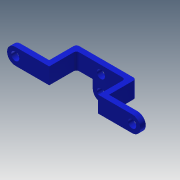
# Autodesk Inventor part: tahlo6
Saved by Autodesk Inventor 2015 (Build 190159000, 159)
## iProperties
Created: 2013-03-23
Part Number: tahlo6
Material: Generic
Document SubType Name: Modeling
Designer: idle-rug
Density: 1 g/cm^3
Appearance: Default
Author: idle-rug
Autodesk Inventor part; units mm, degrees
ref_plane "YZ Plane" through (0, 0, 0) normal (1, 0, 0) x (0, 1, 0)
ref_plane "XZ Plane" through (0, 0, 0) normal (0, 1, 0) x (-1, 0, 0)
ref_plane "XY Plane" through (0, 0, 0) normal (0, 0, 1) x (1, 0, 0)
sketch "Sketch1" plane through (0, 0, 0) normal (0, 1, 0) x (-1, 0, 0)
  line L0 (11, 3) -> (-11, 3)
  line L1 (-11, 3) -> (-11, -3)
  line L2 (-11, -3) -> (11, -3)
  line L3 (11, -3) -> (11, 3)
  line L4 (11, 3) -> (-11, -3) construction
  line L5 (-11, 3) -> (11, -3) construction
  point P0 (0, 0)
  dimension "d0" = 22
  dimension "d1" = 6
  constraints: 12 end point, 2 midpoint, 2 parallel, 1 horizontal, 1 perpendicular
  measures "d0" distance of L2.end L1.end
  measures "d1" distance of L1.end L0.end
extrude "Extrusion1" add sketch "Sketch1" along normal blind 2
sketch "Sketch2" plane through (0, 0, 0) normal (0, -1, 0) x (1, 0, 0)
  line L0 (11, -3) -> (-11, -3) projected
  line L1 (-11, 3) -> (-9, 3)
  line L2 (-9, 3) -> (-9, -3)
  line L3 (-9, -3) -> (-11, -3)
  line L4 (-11, -3) -> (-11, 3)
  line L5 (11, 3) -> (9, 3)
  line L6 (9, 3) -> (9, -3)
  line L7 (9, -3) -> (11, -3)
  line L8 (11, -3) -> (11, 3)
  point P0 (0, 0)
  dimension "d4" = 2
  dimension "d5" = 2
  constraints: 16 end point, 4 parallel, 2 horizontal, 2 perpendicular, 2 point on line
  measures "d4" distance of L2.end L3.end
  measures "d5" distance of L7.end L6.end
extrude "Extrusion2" add sketch "Sketch2" along normal blind 10
sketch "Sketch3" plane through (11, 2, 3) normal (1, 0, 0) x (0, 0, -1)
  line L0 (0, -12) -> (6, -12)
  line L1 (6, -12) -> (6, -10)
  line L2 (6, -10) -> (0, -10)
  line L3 (0, -10) -> (0, -12)
  point P0 (3, -2)
  dimension "d8" = 6
  dimension "d9" = 2
  constraints: 8 end point, 2 parallel, 1 horizontal, 1 perpendicular
  measures "d8" distance of L2.end L1.end
  measures "d9" distance of L1.end L0.end
sketch "Sketch4" plane through (-11, 2, -3) normal (-1, 0, 0) x (0, 0, 1)
  line L0 (0, -12) -> (6, -12)
  line L1 (6, -12) -> (6, -10)
  line L2 (6, -10) -> (0, -10)
  line L3 (0, -10) -> (0, -12)
  point P0 (3, -2)
  dimension "d10" = 6
  dimension "d11" = 2
  constraints: 8 end point, 2 parallel, 1 horizontal, 1 perpendicular
  measures "d10" distance of L2.end L1.end
  measures "d11" distance of L1.end L0.end
extrude "Extrusion3" add sketch "Sketch4" along normal blind 14
extrude "Extrusion4" add sketch "Sketch3" along normal blind 14
sketch "Sketch5" plane through (11, -8, 3) normal (0, 1, 0) x (1, 0, 0)
  line L0 (0, 0) -> (14, 0) projected
  line L1 (14, 6) -> (14, 0) projected
  line L2 (0, 6) -> (14, 6) projected
  line L3 (14, 3) -> (10.5, 3)
  circle A0 centre (10.5, 3) radius 3.5
  line L4 (12.3028, 6) -> (14, 6)
  line L5 (14, 3) -> (14, 6)
  line L6 (14, 3) -> (14, 0)
  line L7 (14, 0) -> (12.3028, 0)
  point P0 (-11, 3)
  dimension "d16" = 3.5
  constraints: 10 end point, 3 collinear, 3 point on circle, 2 point on line, 2 tangent, 1 centre point, 1 coincident, 1 midpoint, 1 parallel
  measures "d16" distance of L3.start L3.end
sketch "Sketch6" plane through (-11, -8, 3) normal (0, 1, 0) x (1, 0, 0)
  line L0 (0, 6) -> (0, 0) projected
  line L1 (0, 6) -> (-14, 6) projected
  line L2 (-14, 0) -> (-14, 6) projected
  line L3 (0, 0) -> (-14, 0) projected
  line L4 (-14, 3) -> (-10.5, 3)
  circle A0 centre (-10.5, 3) radius 3.5
  line L5 (-12.3028, 0) -> (-14, 0)
  line L6 (-14, 0) -> (-14, 3)
  line L7 (-14, 6) -> (-14, 3)
  line L8 (-14, 6) -> (-12.3028, 6)
  point P0 (11, 3)
  point P1 (0, -0.5)
  dimension "d17" = 3.5
  constraints: 10 end point, 3 point on circle, 1 centre point, 1 coincident, 1 horizontal, 1 midpoint, 1 perpendicular, 1 point on line, 2 other
  measures "d17" distance of L4.start L4.end
extrude "Extrusion5" cut sketch "Sketch5" against normal blind 2 contours A0 L1 L0 | A0 L2 L1
extrude "Extrusion6" cut sketch "Sketch6" against normal blind 2 contours A0 L2 L1 | L3 L2 A0
sketch "Sketch7" plane through (11, -8, 3) normal (0, 1, 0) x (1, 0, 0)
  arc A0 (12.3028, 0) -> (12.3028, 6) centre (10.5, 3) ccw projected
  circle A1 centre (10.5, 3) radius 1.5
  point P0 (-11, 3)
  dimension "d22" = 3
  constraints: 1 centre point, 1 coincident
  measures "d22" diameter of A1
extrude "Extrusion7" cut sketch "Sketch7" against normal blind 2
sketch "Sketch8" plane through (-11, -8, 3) normal (0, 1, 0) x (1, 0, 0)
  arc A0 (-12.3028, 6) -> (-12.3028, 0) centre (-10.5, 3) ccw projected
  circle A1 centre (-10.5, 3) radius 1.5
  point P0 (11, 3)
  dimension "d25" = 3
  constraints: 1 centre point, 1 coincident
  measures "d25" diameter of A1
extrude "Extrusion8" cut sketch "Sketch8" against normal blind 2
fillet "Fillet1" radius 1 4 edges at (11, 2, 0) (-11, 2, 0) (9, 0, 0) (-9, 0, 0)
sketch "Sketch9" plane through (0, 2, 0) normal (0, 1, 0) x (1, 0, 0)
  line L0 (-10, -3) -> (10, -3) projected
  line L1 (10, 3) -> (-10, 3) projected
  line L2 (0, -3) -> (0, 0)
  circle A0 centre (0, 0) radius 1.5
  point P0 (0, 0)
  dimension "d29" = 3
  dimension "d30" = 3
  constraints: 2 end point, 1 centre point, 1 coincident, 1 midpoint, 1 perpendicular
  measures "d29" distance of L2.start L2.end
  measures "d30" diameter of A0
extrude "Extrusion9" cut sketch "Sketch9" against normal blind 2
sketch "Sketch10" plane through (0, 2, 0) normal (0, 1, 0) x (1, 0, 0)
  circle A0 centre (0, 0) radius 1.5 projected
  line L0 (10, 3) -> (-10, 3) projected
  line L1 (0, 0) -> (0, 6)
  circle A1 centre (0, 6) radius 1.5
  line L2 (0, 6) -> (0, 9)
  line L3 (-3.5, 5) -> (-3.5, 3)
  line L4 (3.5, 5) -> (3.5, 3)
  arc A2 (3.5, 5) -> (-3.5, 5) centre (0, 5) ccw
  line L5 (-3.5, 3) -> (3.5, 3)
  point P0 (0, 0)
  dimension "d33" = 6
  dimension "d34" = 3
  dimension "d35" = 3
  constraints: 10 end point, 3 perpendicular, 2 centre point, 2 collinear, 2 point on circle, 2 point on line, 2 tangent, 1 coincident
  measures "d33" distance of L1.start L1.end
  measures "d34" diameter of A1
  measures "d35" distance of L2.start L2.end
extrude "Extrusion10" add sketch "Sketch10" against normal blind 2 contours L0 L3 A2 L2 A1 L1 | L1 A1 L2 A2 L4 L0
sketch "Sketch11" plane through (11, -8, 3) normal (0, 1, 0) x (1, 0, 0)
  arc A0 (12.3028, 0) -> (12.3028, 6) centre (10.5, 3) ccw projected
  line L0 (0, 6) -> (12.3028, 6) projected
  line L1 (0, 0) -> (12.3028, 0) projected
  circle A1 centre (10.5, 3) radius 3
  line L2 (10.5, 0) -> (12.3028, 0)
  line L3 (10.5, 6) -> (12.3028, 6)
  arc A2 (12.3028, 0) -> (12.3028, 6) centre (10.5, 3) ccw
  point P0 (-11, 3)
  constraints: 4 end point, 4 point on circle, 4 tangent, 2 centre point, 2 collinear, 2 point on line, 1 coincident
extrude "Extrusion11" cut sketch "Sketch11" against normal blind 2 contours L1 A1 L0 A0
sketch "Sketch12" plane through (-11, -8, 3) normal (0, 1, 0) x (1, 0, 0)
  arc A0 (-12.3028, 6) -> (-12.3028, 0) centre (-10.5, 3) ccw projected
  line L0 (0, 0) -> (-12.3028, 0) projected
  line L1 (0, 6) -> (-12.3028, 6) projected
  circle A1 centre (-10.5, 3) radius 3
  line L2 (-12.3028, 0) -> (-10.5, 0)
  line L3 (-12.3028, 6) -> (-10.5, 6)
  arc A2 (-12.3028, 6) -> (-12.3028, 0) centre (-10.5, 3) ccw
  point P0 (11, 3)
  constraints: 4 end point, 4 point on circle, 2 centre point, 2 point on line, 2 tangent, 1 coincident
extrude "Extrusion12" cut sketch "Sketch12" against normal blind 2 contours L1 A1 L0 A0
sketch "Sketch13" plane through (0, 2, 0) normal (0, 1, 0) x (1, 0, 0)
  circle A0 centre (0, 6) radius 1.5 projected
  line L0 (3.5, 3) -> (3.5, 5) projected
  arc A1 (3.5, 5) -> (-3.5, 5) centre (0, 5) ccw projected
  line L1 (-3.5, 5) -> (-3.5, 3) projected
  line L2 (-3.5, 3) -> (-10, 3) projected
  circle A2 centre (0, 6) radius 1.5
  circle A3 centre (0, 6) radius 3
  line L3 (-3.5, 3) -> (3.5, 3)
  line L4 (3.5, 3) -> (3.5, 5)
  line L5 (-3.5, 3) -> (-3.5, 5)
  line L6 (-3, 6) -> (-3, 3)
  line L7 (3, 6) -> (3, 3)
  line L8 (-3, 3) -> (-3.5, 3)
  line L9 (3, 3) -> (3.5, 3)
  arc A4 (3.5, 5) -> (-3.5, 5) centre (0, 5) ccw
  dimension "d44" = 3
  dimension "d45" = 6
  constraints: 14 end point, 6 tangent, 5 collinear, 4 point on circle, 3 centre point, 2 coincident, 2 perpendicular, 2 point on line
  measures "d44" diameter of A2
  measures "d45" diameter of A3
extrude "Extrusion13" cut sketch "Sketch13" against normal blind 2 contours L3 L7 A3 A1 L0 | A3 A1 | A3 L6 L3 L1 A1 picked at (-2.1113, 7.1747)
sketch "Sketch14" plane through (0, 2, 0) normal (0, 1, 0) x (1, 0, 0)
  arc A0 (-3, 6) -> (3, 6) centre (0, 6) ccw projected
  circle A1 centre (0, 6) radius 3
  circle A2 centre (0, 6) radius 1.5
  dimension "d48" = 3
  constraints: 2 centre point, 2 coincident, 1 concentric
  measures "d48" diameter of A2
extrude "Extrusion14" add sketch "Sketch14" against normal blind 2
body "Solid1"
